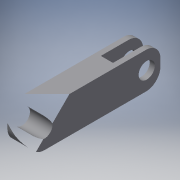
# Autodesk Inventor part: lever2
Saved by Autodesk Inventor 2016 (Build 200138000, 138)
## iProperties
Created: 2015-09-30
Part Number: lever2
Material: Generic
Document SubType Name: Modeling
Designer: Jesse Stevenson
Density: 1 g/cm^3
Appearance: Default
Author: Jesse Stevenson
Autodesk Inventor part; units mm, degrees
ref_plane "YZ Plane" through (0, 0, 0) normal (1, 0, 0) x (0, 1, 0)
ref_plane "XZ Plane" through (0, 0, 0) normal (0, 1, 0) x (-1, 0, 0)
ref_plane "XY Plane" through (0, 0, 0) normal (0, 0, 1) x (1, 0, 0)
ref_plane "Work Plane1" through (8.001, 26.0985, -18.0717) normal (0, 1, 0) x (0, 0, -1)
sketch "Sketch1" plane through (8.001, 26.0985, -18.0717) normal (0, 1, 0) x (0, 0, -1)
  line L0 (-18.0717, -2.667) -> (-9.319, -2.667) projected
  line L1 (-9.319, 0) -> (-18.0717, 0) projected
  line L2 (-9.319, -2.667) -> (-18.0717, -2.667)
  line L3 (-18.0717, -2.667) -> (-18.0717, 0) construction
  line L4 (-18.0717, 0) -> (-9.319, 0)
  line L5 (-9.319, 0) -> (-9.319, -2.667) construction
  line L6 (-9.319, -2.667) -> (-23.6934, -2.667)
  line L7 (-40.2342, -2.667) -> (-40.2342, -3.8142)
  line L8 (-40.2342, -3.8142) -> (-9.319, -3.8142)
  line L9 (-9.319, -3.8142) -> (-9.319, -2.667)
  line L10 (-9.319, 0) -> (-23.6934, 0)
  line L11 (-40.2342, 0) -> (-40.2342, 1.1472)
  line L12 (-40.2342, 1.1472) -> (-9.319, 1.1472)
  line L13 (-9.319, 1.1472) -> (-9.319, 0)
  line L14 (-23.6934, -2.667) -> (-23.6934, 0)
  line L15 (-40.2342, -2.667) -> (-40.2342, 0)
  point P0 (-18.0717, 8.001)
  constraints: 28 end point, 6 parallel, 4 perpendicular, 3 horizontal, 2 collinear
extrude "Extrusion1" add sketch "Sketch1" along normal blind 7.9375
sketch "Sketch2" plane through (11.8152, 26.0985, 22.1625) normal (1, 0, 0) x (0, 0, -1)
  line L0 (0, 0) -> (30.9152, 0) construction
  line L1 (30.9152, 0) -> (30.9152, 7.9375) construction
  line L2 (0, 7.9375) -> (30.9152, 7.9375) construction
  line L3 (0, 0) -> (0, 7.9375) construction
  line L4 (30.9152, 0) -> (30.9152, 7.9375) construction
  line L5 (30.9152, 3.9687) -> (0, 3.9687) construction
  line L6 (0, 0) -> (30.9152, 0) construction
  line L7 (25.6796, 0) -> (25.6796, 7.9375) construction
  line L8 (30.9152, 7.9375) -> (16.5409, 7.9375) construction
  circle A0 centre (25.6796, 3.9687) radius 1.7859
  point P0 (22.1625, -26.0985)
  dimension "d8" = 3.5719
  constraints: 4 end point, 3 midpoint, 2 point on line, 1 centre point, 1 perpendicular
  measures "d8" diameter of A0
extrude "Extrusion2" cut sketch "Sketch2" against normal through all
fillet "Fillet1" radius 3.175 2 edges at (9.3345, 34.036, 22.1625) (9.3345, 26.0985, 22.1625)
sketch "Sketch3" plane through (11.8152, 26.0985, -8.7527) normal (1, 0, 0) x (0, 0, -1)
  circle A0 centre (-5.2356, 3.9688) radius 1.7859 projected
  arc A1 (-30.9152, 3.175) -> (-27.7402, 0) centre (-27.7402, 3.175) ccw projected
  line L0 (-27.7402, 0) -> (0, 0) projected
  line L1 (0, 0) -> (0, 7.9375) projected
  line L2 (-27.7402, 7.9375) -> (0, 7.9375) projected
  arc A2 (-27.7402, 7.9375) -> (-30.9152, 4.7625) centre (-27.7402, 4.7625) ccw projected
  line L3 (-30.9152, 3.175) -> (-30.9152, 4.7625) projected
  line L4 (-27.7402, 3.175) -> (-27.7402, 4.7625) construction
  circle A3 centre (-27.7402, 3.9687) radius 1.7859
  point P0 (-8.7527, -26.0985)
  dimension "d7" = 3.5719
  constraints: 2 end point, 1 centre point, 1 midpoint, 1 vertical
  measures "d7" diameter of A3
extrude "Extrusion3" cut sketch "Sketch3" against normal through all contours A3
sketch "Sketch5" plane through (11.8152, 26.0985, -8.7527) normal (1, 0, 0) x (0, 0, -1)
  circle A0 centre (-27.7402, 3.9688) radius 1.7859 construction
  circle A1 centre (-5.2356, 3.9688) radius 1.7859 construction
  arc A2 (-30.9152, 3.175) -> (-27.7402, 0) centre (-27.7402, 3.175) ccw construction
  line L0 (-27.7402, 0) -> (0, 0) construction
  line L1 (0, 0) -> (0, 7.9375) construction
  line L2 (-27.7402, 7.9375) -> (0, 7.9375) construction
  arc A3 (-27.7402, 7.9375) -> (-30.9152, 4.7625) centre (-27.7402, 4.7625) ccw construction
  line L3 (-30.9152, 3.175) -> (-30.9152, 4.7625) construction
  line L4 (-14.3743, 0) -> (0, 0) projected
  line L5 (-2.2351, 0) -> (-2.2351, 7.9375)
  line L6 (-14.3743, 7.9375) -> (0, 7.9375) projected
  line L7 (-2.2351, 0) -> (-8.7527, 0)
  line L8 (-27.7402, 7.9375) -> (0, 7.9375) projected
  line L9 (-2.2351, 0) -> (0, 0)
  line L10 (0, 0) -> (0, 7.9375)
  line L11 (0, 7.9375) -> (-2.2351, 7.9375)
  line L12 (-2.2351, 7.9375) -> (-2.2351, 0)
  point P0 (-8.7527, -26.0985)
  constraints: 12 end point, 3 point on line, 2 parallel, 2 perpendicular, 1 horizontal
extrude "Extrusion4" cut sketch "Sketch5" against normal through all
fillet "Fillet2" radius 3.175 4 edges at (11.2416, 34.036, -6.5176) (7.4274, 34.036, -6.5176) (11.2416, 26.0985, -6.5176) (7.4274, 26.0985, -6.5176)
body "Solid1"
